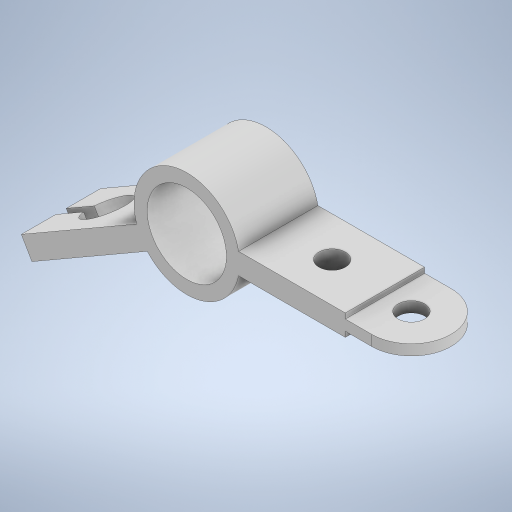
# Autodesk Inventor part: Pieza1-Tarea1
Saved by Autodesk Inventor 2024 (Build 280153000, 153)
## iProperties
Created: 2024-02-16
Part Number: Pieza1-Tarea1
Material: Genérico
Document SubType Name: Modeling
Designer: Diegolap
Mass: 9.68856 g
Surface Area: 65.0856 cm^2
Volume: 9.68856 cm^3
Density: 1 g/cm^3
Appearance: Valor por defecto
Author: Diegolap
Autodesk Inventor part; units mm, degrees
ref_plane "YZ Plane" through (0, 0, 0) normal (1, 0, 0) x (0, 1, 0)
ref_plane "XZ Plane" through (0, 0, 0) normal (0, 1, 0) x (-1, 0, 0)
ref_plane "XY Plane" through (0, 0, 0) normal (0, 0, 1) x (1, 0, 0)
sketch "Boceto1" plane through (0, 0, 0) normal (0, 0, 1) x (1, 0, 0)
  circle A0 centre (0, 0) radius 9.525
  line L0 (12.4434, -2.54) -> (38.1, -2.54)
  line L1 (38.1, -2.54) -> (38.1, 2.54)
  line L2 (38.1, 2.54) -> (12.4434, 2.54)
  line L3 (12.7, 0) -> (9.5196, 0.3221) construction
  line L4 (9.5196, -0.3221) -> (12.7, 0) construction
  line L5 (-9.5063, -8.4214) -> (-37.2364, -24.4314)
  line L6 (-37.2364, -24.4314) -> (-39.7764, -20.032)
  line L7 (-39.7764, -20.032) -> (-12.0463, -4.022)
  line L8 (0.4725, -1.9521) -> (-1.0609, -2.54) construction
  arc A1 (12.4434, 2.54) -> (-12.0463, -4.022) centre (0, 0) ccw
  arc A2 (-9.5063, -8.4214) -> (12.4434, -2.54) centre (0, 0) ccw
  line L9 (38.1, -1.27) -> (44.45, -1.27)
  line L10 (44.45, -1.27) -> (44.45, 1.27)
  line L11 (44.45, 1.27) -> (38.1, 1.27)
  point P0 (-23.3714, -16.4264)
  point P1 (-38.5064, -22.2317)
  point P2 (41.275, -1.27)
  point P3 (41.275, 1.27)
  dimension "d0" = 19.05
  dimension "d3" = 5.08
  dimension "d4" = 2.54
  dimension "d7" = 5.08
  dimension "d8" = 38.5064
  dimension "d9" = 2.54
  dimension "d10" = 44.4634
  dimension "d11" = 3.175
  dimension "d12" = 3.175
  dimension "d13" = 38.1
  dimension "d14" = 6.35
  dimension "d16" = 2.54
  dimension "d17" = 1.27
  constraints: 24 end point, 6 point on circle, 4 midpoint, 3 centre point, 3 parallel, 3 perpendicular, 3 point on line, 2 coincident, 2 horizontal
  measures "d0" diameter of A0
  measures "d3" distance between parallel lines of L2 L0
  measures "d4" distance from line of A0.centre L2
  measures "d7" distance from line of point (-23.371, -16.426) L7
  measures "d8" horizontal distance of point (0, 0) point (-38.506, -22.232)
  measures "d9" distance from line of L7 A0.centre
  measures "d10" distance from line of A0.centre L6
  measures "d11" radial gap between concentric circles of A0 A1
  measures "d12" radial gap between concentric circles of A0 A2
  measures "d13" distance from line of A0.centre L1
  measures "d14" distance between parallel lines of L1 L10
  measures "d16" distance of point (41.275, -1.27) point (41.275, 1.27)
  measures "d17" distance between parallel lines of L2 L11
extrude "Extrusión1" add sketch "Boceto1" along normal blind 19.05
sketch "Boceto2" plane through (38.1, 1.27, 0) normal (0, 1, 0) x (1, 0, 0)
  line L0 (6.35, 0) -> (0, 0) projected
  line L1 (6.35, -19.05) -> (0, -19.05) projected
  line L2 (6.35, 0) -> (6.35, -19.05)
  arc A0 (6.35, -19.05) -> (6.35, 0) centre (6.35, -9.525) ccw
  point P0 (-38.1, 0)
  constraints: 2 end point, 2 point on circle, 2 tangent, 1 centre point, 1 vertical
extrude "Extrusión2" add sketch "Boceto2" against normal blind 2.54
sketch "Boceto3" plane through (38.1, 1.27, 19.05) normal (0, 1, 0) x (1, 0, 0)
  line L0 (0, 19.05) -> (0, 0) projected
  line L1 (0, 19.05) -> (0, 9.525)
  line L2 (0, 19.05) -> (6.35, 19.05) projected
  line L3 (0, 0) -> (6.35, 0) projected
  line L4 (6.35, 19.05) -> (6.35, 0)
  line L5 (6.35, 0) -> (6.35, 9.525)
  circle A0 centre (6.35, 9.525) radius 3.175
  point P0 (-38.1, 19.05)
  dimension "d22" = 6.35
  constraints: 6 end point, 2 midpoint, 1 centre point, 1 coincident, 1 vertical
  measures "d22" diameter of A0
extrude "Extrusión3" cut sketch "Boceto3" against normal blind 2.54 contours A0 L4 | L4 A0
sketch "Boceto4" plane through (12.4434, 2.54, 0) normal (0, 1, 0) x (1, 0, 0)
  line L0 (25.7224, -0.5661) -> (25.7224, -18.5033)
  line L1 (25.7224, -18.5033) -> (25.6566, -9.525)
  line L2 (25.6566, 0) -> (25.6566, -19.05) projected
  line L3 (25.6566, -9.525) -> (12.9566, -9.525)
  circle A0 centre (12.9566, -9.525) radius 3.175
  point P0 (-12.4434, 0)
  dimension "d25" = 12.7
  dimension "d26" = 6.35
  constraints: 6 end point, 1 centre point, 1 coincident, 1 horizontal, 1 midpoint, 1 vertical
  measures "d25" distance of L1.end L3.end
  measures "d26" diameter of A0
extrude "Extrusión4" cut sketch "Boceto4" against normal blind 5.08
sketch "Boceto5" plane through (-39.7764, -20.032, 19.05) normal (-0.5, 0.866, 0) x (0.866, 0.5, 0)
  line L0 (0, 19.05) -> (0, 0) projected
  line L1 (0, 0) -> (0, 19.05)
  line L2 (0, 19.05) -> (0, 9.525)
  line L3 (0, 9.525) -> (12.7, 9.525)
  circle A0 centre (12.7, 9.525) radius 5.08
  line L4 (7.7813, 8.255) -> (0, 8.255)
  line L5 (0, 8.255) -> (0, 10.795)
  line L6 (0, 10.795) -> (7.7813, 10.795)
  point P0 (44.4634, 19.05)
  point P1 (6.35, 9.525)
  point P2 (0, 10.795)
  point P3 (0, 8.255)
  dimension "d29" = 12.7
  dimension "d30" = 10.16
  dimension "d31" = 1.27
  dimension "d32" = 1.27
  constraints: 12 end point, 2 midpoint, 2 parallel, 2 point on circle, 1 centre point, 1 coincident, 1 collinear, 1 horizontal, 1 perpendicular
  measures "d29" distance of L2.end L3.end
  measures "d30" diameter of A0
  measures "d31" distance between parallel lines of L6 L3
  measures "d32" distance from line of point (6.35, 9.525) L4
extrude "Extrusión5" cut sketch "Boceto5" against normal blind 5.08
